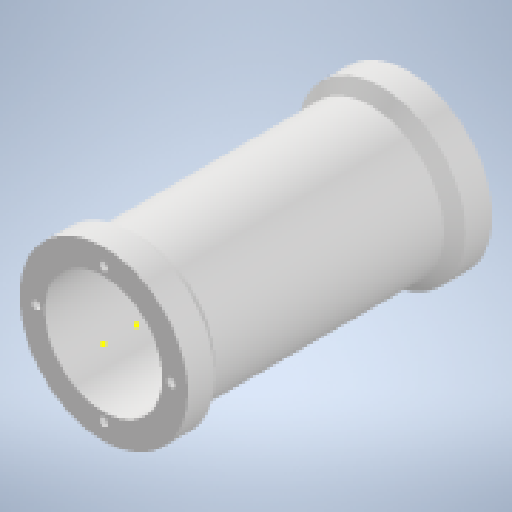
# Autodesk Inventor part: korpus
Saved by Autodesk Inventor 2025 (Build 290162000, 162)
## iProperties
Created: 2025-03-15
Part Number: korpus
Material: Ogólny
Document SubType Name: Modeling
Designer: barte
Density: 1 g/cm^3
Appearance: Domyślna
Author: barte
Autodesk Inventor part; units mm, degrees
ref_plane "YZ Plane" through (0, 0, 0) normal (1, 0, 0) x (0, 1, 0)
ref_plane "XZ Plane" through (0, 0, 0) normal (0, 1, 0) x (-1, 0, 0)
ref_plane "XY Plane" through (0, 0, 0) normal (0, 0, 1) x (1, 0, 0)
sketch "Szkic1" plane through (0, 0, 0) normal (1, 0, 0) x (0, 1, 0)
  point P0 (0, 0)
sketch "Szkic2" plane through (0, 0, 0) normal (1, 0, 0) x (0, 1, 0)
  point P0 (0, 0)
sketch "Szkic3" plane through (0, 0, 0) normal (1, 0, 0) x (0, 1, 0)
  line L0 (0, 19.7455) -> (50, 19.7455)
  line L1 (50, 19.7455) -> (50, 3.5455)
  line L2 (50, 3.5455) -> (43.564, -2.8878)
  line L3 (43.564, -2.8878) -> (43.564, -138.8878)
  line L4 (43.564, -138.8878) -> (50, -145.3212)
  line L5 (50, -145.3212) -> (50, -161.5212)
  line L6 (50, -161.5212) -> (0, -161.5212)
  line L7 (0, 19.7455) -> (0, -161.5212)
  point P0 (0, 0)
  dimension "d0" = 50
  dimension "d1" = 16.2
  dimension "d2" = 9.1
  dimension "d3" = 136
  dimension "d4" = 9.1
  dimension "d5" = 16.2
  constraints: 16 end point, 4 vertical, 2 horizontal
  measures "d0" distance of L0.start L0.end
  measures "d1" distance of L0.end L1.end
  measures "d2" distance of L1.end L2.end
  measures "d3" distance of L2.end L3.end
  measures "d4" distance of L3.end L4.end
  measures "d5" distance of L4.end L5.end
revolve "Obrót1" add sketch "Szkic3" angle 360 about axis through (0, 0, 19.7455) along (0, 0, -1)
sketch "Szkic4" plane through (0, 0, -161.5212) normal (0, 0, -1) x (-1, 0, 0)
  line L0 (0, 0) -> (40, 0)
  line L1 (0, 0) -> (0, -40)
  line L2 (0, 0) -> (-40, 0)
  line L3 (0, 0) -> (0, 40)
  dimension "d7" = 40
  dimension "d8" = 40
  dimension "d9" = 40
  dimension "d10" = 40
  constraints: 8 end point, 2 horizontal, 2 vertical
  measures "d7" distance of L0.start L0.end
  measures "d8" distance of L0.start L1.end
  measures "d9" distance of L0.start L2.end
  measures "d10" distance of L0.start L3.end
hole "Otwór1" at (0, 40, -161.5212) at (-40, 0, -161.5212) at (0, -40, -161.5212) at (40, 0, -161.5212) direction (0, 0, 1) diameter 5 depth 18.5 tip angle 118
sketch "Szkic5" plane through (0, 0, 19.7455) normal (0, 0, 1) x (1, 0, 0)
  circle A0 centre (40, 0) radius 2.5 projected
  line L0 (0, 0) -> (40, 0)
  circle A1 centre (0, -40) radius 2.5 projected
  line L1 (0, 0) -> (0, -40)
  circle A2 centre (0, 0) radius 50 projected
  circle A3 centre (-40, 0) radius 2.5 projected
  line L2 (0, 0) -> (-40, 0)
  circle A4 centre (0, 40) radius 2.5 projected
  line L3 (0, 0) -> (0, 40)
  constraints: 8 end point, 2 horizontal, 2 vertical
hole "Otwór2" at (-40, 0, 19.7455) at (0, 40, 19.7455) at (40, 0, 19.7455) at (0, -40, 19.7455) direction (0, 0, -1) diameter 5 depth 18.5 tip angle 118
sketch "Szkic6" plane through (0, 0, 19.7455) normal (0, 0, 1) x (1, 0, 0)
  line L0 (0, 0) -> (0, 50)
  circle A0 centre (0, 0) radius 50 projected
  constraints: 2 end point, 1 vertical, 1 vertical alignment, 1 other
hole "Otwór3" at (0, 0, 19.7455) direction (0, 0, -1) diameter 70 end through all
sketch "Szkic7" plane through (0, 0, 19.7455) normal (0, 0, 1) x (1, 0, 0)
  point P0 (0, 0)
